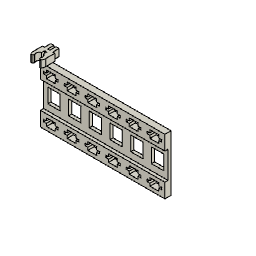
3mmビットホルダ v2 (Autodesk Fusion 360 design; units mm, degrees)
Autodesk Fusion 360 part; units mm, degrees
sketch "スケッチ1" plane through (0, 0, 0) normal (0, 0, 1) x (1, 0, 0)
  line L0 (-0.5, 1.519868) -> (-0.5, 3.5)
  line L1 (0.5, 3.5) -> (0.5, 1.519868)
  line L2 (-3, 0) -> (-3, 3.487815)
  line L3 (-1.811769, 6.5) -> (1.811769, 6.5)
  line L4 (3, 3.487815) -> (3, 0)
  line L5 (-0.5, 3.5) -> (0.5, 3.5)
  line L6 (1.02846, -1.225671) -> (1.928363, -2.298133)
  line L7 (0, 0) -> (3.962322, 0) construction
  line L8 (0, 0) -> (0, 0.7)
  line L9 (-1.02846, -1.225671) -> (-1.928363, -2.298133)
  arc A0 (-0.5, 1.519868) -> (-1.02846, -1.225671) centre (0, 0) ccw
  arc A1 (1.02846, -1.225671) -> (0.5, 1.519868) centre (0, 0) ccw
  arc A2 (-3, 0) -> (-1.928363, -2.298133) centre (0, 0) ccw
  arc A3 (1.928363, -2.298133) -> (3, 0) centre (0, 0) ccw
  line L10 (-1.811769, 3.487815) -> (-1.811769, 6.5)
  line L11 (1.811769, 3.487815) -> (1.811769, 6.5)
  line L12 (1.811769, 3.487815) -> (3, 3.487815)
  line L13 (-3, 3.487815) -> (-1.811769, 3.487815)
  line L14 (-0.5, 3.487815) -> (0.5, 3.487815)
  dimension "d1" = 3.2
  dimension "d4" = 6
  dimension "d6" = 50
  constraint coincident L7.start L8.start
  constraint concentric A0 A2
  constraint tangent L2 A2
  constraint perpendicular L2 L3
  constraint tangent L4 A2
  constraint perpendicular L3 L4
  constraint perpendicular L1 L5
  constraint horizontal L7
  constraint perpendicular L7 L8
  constraint concentric A0 A1
  constraint concentric A2 A3
  constraint perpendicular L4 L13
  constraint perpendicular L3 L10
  constraint collinear L12 L13
  constraint collinear L13 L14
  measures "d1" diameter of A0
  measures "d4" diameter of A2
  measures "d6" angle of L6 L7
extrude "押し出し1" add sketch "スケッチ1" along normal blind 3 contours L0 L1 L2 L3 L4 L5 L6 L9 A0 A1 A2 A3 L10 L11 L12 L13 picked at (0.166667, 5.5) makes body 1
sketch "スケッチ2" plane through (0, 6.5, 0) normal (0, 1, 0) x (-1, 0, 0)
  line L0 (-1.811769, 0) -> (1.811769, 0)
  line L1 (1.811769, 0) -> (1.811769, 3)
  line L2 (1.811769, 3) -> (-1.811769, 3)
  line L3 (-1.811769, 3) -> (-1.811769, 0)
  line L4 (-5, -2.005016) -> (5, -2.005016)
  line L5 (5, -2.005016) -> (5, 5)
  line L6 (5, 5) -> (-5, 5)
  line L7 (-5, 5) -> (-5, -2.005016)
  constraint horizontal L4
  constraint vertical L5
  constraint horizontal L6
  constraint vertical L7
extrude "押し出し2" add sketch "スケッチ2" against normal blind 3 separate body contours L4 L5 L6 L7 picked at (-3.937256, 0.998328) makes body 2
copy_body "ボディのコピーと貼り付け1" bodies 2 makes body 3
move_body "移動1" bodies 3 to x (1, 0, 0) y (0, 1, 0) z (0, 0, 1) at (0, 0, -30)
delete_body "RemoveBody1" bodies 3
move_face "面を移動1" by (0, 0, 0.3) 1 faces at (0.603923, 4.5, 3) on bodies 2
move_face "面を移動2" by (0.3, 0, 0) 1 faces at (1.811769, 5.5, 2.2) on bodies 2
move_face "面を移動3" by (-0.3, 0, 0) 1 faces at (-1.811769, 5.5, 1.1) on bodies 2
move_face "面を移動4" by (0, 0, -0.3) 1 faces at (0.703923, 5.5, 0) on bodies 2
sketch "スケッチ3" plane through (0, 6.5, 0) normal (0, 1, 0) x (-1, 0, 0)
  line L0 (-2.111769, -0.3) -> (-2.111769, 3.3)
  line L1 (-2.111769, 3.3) -> (2.111769, 3.3)
  line L2 (2.111769, 3.3) -> (2.111769, -0.3)
  line L3 (2.111769, -0.3) -> (-2.111769, -0.3)
  line L4 (-5, 5) -> (-5, -2.005016)
  line L5 (-5, -2.005016) -> (5, -2.005016)
  line L6 (5, -2.005016) -> (5, 5)
  line L7 (5, 5) -> (-5, 5)
  line L8 (3.5, 1) -> (-3.5, 1)
  line L9 (-3.5, 1) -> (-3.5, 2)
  line L10 (-3.5, 2) -> (3.5, 2)
  line L11 (3.5, 2) -> (3.5, 1)
  line L12 (3.5, 1) -> (-3.5, 2) construction
  line L13 (-3.5, 1) -> (3.5, 2) construction
  point P0 (0, 1.5)
  dimension "d11" = 7
  dimension "d12" = 1
  constraint horizontal L8
  constraint perpendicular L8 L9
  constraint parallel L8 L10
  constraint parallel L9 L11
  constraint coincident L12 P0
  constraint coincident L13 P0
  measures "d11" distance of L9.end L10.end
  measures "d12" distance of L8.end L9.end
extrude "押し出し3" cut sketch "スケッチ3" against normal blind 3.7 contours L0 L8 L9 L10 | L2 L8 L10 L11 picked at (-2.574513, 1.333333) picked at (2.574513, 1.666667) bodies 2
copy_body "ボディのコピーと貼り付け2" bodies 2 makes body 4
move_body "移動2" bodies 4 to x (1, 0, 0) y (0, 1, 0) z (0, 0, 1) at (0, 0, -30)
sketch "スケッチ4" plane through (0, 0, -2.005016) normal (0, 0, -1) x (1, 0, 0)
  line L0 (-5, -6.5) -> (5, -6.5)
  line L1 (5, -6.5) -> (5, -3.5)
  line L2 (5, -3.5) -> (-5, -3.5)
  line L3 (-5, -3.5) -> (-5, -6.5)
  line L4 (-5, -5) -> (5, -5)
  constraint midpoint L3 L4.start
  constraint midpoint L1 L4.end
extrude "押し出し4" add sketch "スケッチ4" along normal blind 23 contours L0 L1 L3 L4 picked at (-1.666667, -5.5) bodies 4 2
sketch "スケッチ5" plane through (0, 5, 0) normal (0, -1, 0) x (1, 0, 0)
  line L0 (-5, -25) -> (5, -25)
  line L1 (5, -25) -> (5, -2.005016)
  line L2 (5, -2.005016) -> (-5, -2.005016)
  line L3 (-5, -2.005016) -> (-5, -25)
  line L4 (2, -22) -> (-1.910963, -22)
  line L5 (-1.910963, -22) -> (-1.910963, -5.005015)
  line L6 (-1.910963, -5.005015) -> (2, -5.005015)
  line L7 (2, -5.005015) -> (2, -22)
  line L8 (2, -22) -> (-1.910963, -5.005015) construction
  line L9 (-1.910963, -22) -> (2, -5.005015) construction
  point P0 (0.044518, -13.502508)
  constraint horizontal L4
  constraint perpendicular L4 L5
  constraint parallel L4 L6
  constraint parallel L5 L7
extrude "押し出し5" cut sketch "スケッチ5" against normal blind 6 contours L4 L5 L6 L7 picked at (0.696346, -16.335005) bodies 4
move_face "面を移動5" by (0, 2, 0) 3 faces at (0.603923, 6.5, 2) (2.207846, 3.487815, 1) (-2.603923, 3.487815, 1) on bodies 1
move_body "移動3" bodies 1 to x (1, 0, 0) y (0, 1, 0) z (0, 0, 1) at (0, -2, 0)
move_face "面を移動6" by (1, 0, 0) 1 faces at (5, 5, -29.67001) on bodies 4
move_face "面を移動7" by (-1, 0, 0) 1 faces at (-5, 5, -29.67001) on bodies 4
move_face "面を移動8" by (-1, 0, 0) 1 faces at (-1.910963, 5.5, -16.335005) on bodies 4
move_face "面を移動9" by (1, 0, 0) 1 faces at (2, 6, -10.67001) on bodies 4
pattern_linear "R パターン1" count 1 spacing 0 along (0, 0, -1) count 6 spacing 12 along (1, 0, 0) of bodies 4 makes body 5 at (12.733602, 6.5, -3.436677) makes body 6 at (24.733602, 6.5, -3.436677) makes body 7 at (36.733602, 6.5, -3.436677) makes body 8 at (48.733602, 6.5, -3.436677) makes body 9 at (60.733602, 6.5, -3.436677)
combine "結合1" operation add target body 4 tool bodies 5 6 7 8 9
copy_body "ボディのコピーと貼り付け3" bodies 4 makes body 10
move_body "移動4" bodies 10 to x (1, 0, 0) y (0, 1, 0) z (0, 0, 1) at (75, 0, 0)
ref_plane "作業平面1" through (81.089037, 5.75, -13.502508) normal (1, 0, 0) x (0, 0, -1)
split "分割1" by plane through (81.089037, 5.75, -13.502508) normal (1, 0, 0) bodies 10 makes body 11 at (92.029679, 6.5, -10.67001)
sketch "スケッチ6" plane through (0, 0, 3) normal (0, 0, 1) x (-1, 0, 0)
  arc A0 (3, 2) -> (1.928363, 4.298133) centre (0, 2) ccw
  line L0 (1.928363, 4.298133) -> (1.02846, 3.225671)
  arc A1 (0.5, 0.480132) -> (1.02846, 3.225671) centre (0, 2) ccw
  line L1 (0.5, 0.480132) -> (0.5, -1.5)
  line L2 (0.5, -1.5) -> (-0.5, -1.5)
  line L3 (-0.5, -1.5) -> (-0.5, 0.480132)
  arc A2 (-1.02846, 3.225671) -> (-0.5, 0.480132) centre (0, 2) ccw
  line L4 (-1.02846, 3.225671) -> (-1.928363, 4.298133)
  arc A3 (-1.928363, 4.298133) -> (-3, 2) centre (0, 2) ccw
  line L5 (-3, 2) -> (-3, -3.487815)
  line L6 (-3, -3.487815) -> (-1.811769, -3.487815)
  line L7 (-1.811769, -3.487815) -> (-1.811769, -6.5)
  line L8 (-1.811769, -6.5) -> (1.811769, -6.5)
  line L9 (1.811769, -6.5) -> (1.811769, -3.487815)
  line L10 (1.811769, -3.487815) -> (3, -3.487815)
  line L11 (3, -3.487815) -> (3, 2)
  line L12 (-0.5, -3.5) -> (0.5, -3.5)
  line L13 (0.5, -3.5) -> (0.5, -9.5)
  line L14 (0.5, -9.5) -> (-0.5, -9.5)
  line L15 (-0.5, -9.5) -> (-0.5, -3.5)
  line L16 (-0.5, -3.5) -> (0.5, -9.5) construction
  line L17 (0.5, -3.5) -> (-0.5, -9.5) construction
  point P0 (0, -6.5)
  constraint horizontal L12
  constraint perpendicular L12 L13
  constraint parallel L12 L14
  constraint parallel L13 L15
  constraint coincident L16 P0
  constraint coincident L17 P0
  constraint midpoint L8 P0
extrude "押し出し6" cut sketch "スケッチ6" against normal blind 6 contours L8 L12 L13 L15 picked at (-0.166667, -4.5) bodies 1
move_body "移動5" bodies 10 to x (1, 0, 0) y (0, 1, 0) z (0, 0, 1) at (-75, 0, 0)
move_face "面を移動10" by (1, 0, 0) 1 faces at (-6, 5, -29.67001) on bodies 10
move_face "面を移動11" by (-1, 0, 0) 1 faces at (6.089037, 5, -29.67001) on bodies 10
copy_body "ボディのコピーと貼り付け4" bodies 10 makes body 12
pattern_linear "R パターン2" count 6 spacing 10 along (1, 0, 0) of bodies 12 makes body 13 at (10.733602, 6.5, -3.436677) makes body 14 at (20.733602, 6.5, -3.436677) makes body 15 at (30.733602, 6.5, -3.436677) makes body 16 at (40.733602, 6.5, -3.436677) makes body 17 at (50.733602, 6.5, -3.436677)
combine "結合2" operation add target body 17 tool bodies 16 15 14 12 13
move_face "面を移動12" by (0.229813, 0.192836, 0) 1 faces at (1.328428, -3.583159, 1) on bodies 1
move_face "面を移動13" by (-0.229813, 0.192836, 0) 1 faces at (-1.328428, -3.583159, 1) on bodies 1
move_face "面を移動14" by (-0.3, 0, 0) 1 faces at (-1.811769, 4.491877, 1) on bodies 1
move_face "面を移動15" by (0.3, 0, 0) 1 faces at (1.811769, 4.491877, 1) on bodies 1
move_face "面を移動16" by (0, 0, 0.4) 1 faces at (-2.422319, 0.154988, 3) on bodies 1
chamfer "面取り1" distance 0.2 angle 45 2 edges at (1.240033, -3.011097, 1.7) (-1.240033, -3.011097, 1.7) on bodies 1
chamfer "面取り2" distance 0.5 angle 45 2 edges at (2.14851, -4.093778, 1.7) (-2.14851, -4.093778, 1.7) on bodies 1
move_face "面を移動17" by (-0.1, 0, 0) 1 faces at (2.111769, 4.491877, 1.133333) on bodies 1
move_face "面を移動18" by (0.1, 0, 0) 1 faces at (-2.111769, 4.491877, 1.133333) on bodies 1
ref_plane "作業平面2" through (25.044518, 5, -13) normal (0, 0, 1) x (-1, 0, 0)
split "分割2" by plane through (25.044518, 5, -13) normal (0, 0, 1) bodies 17 makes body 18 at (0.733602, 6.5, -3.436677)
move_body "移動6" bodies 18 to x (1, 0, 0) y (0, 1, 0) z (0, 0, 1) at (0, 0, -10)
combine "結合3" operation add target body 17 tool bodies 18
delete_body "RemoveBody2" bodies 11
delete_body "RemoveBody3" bodies 4
delete_body "RemoveBody4" bodies 10
move_face "面を移動19" by (0, -1, 0) 5 faces at (1.003923, 6.5, 1.133333) (-1.507846, 6.5, 1.133333) (-0.166667, 3.5, 1.133333) (2.34118, 3.487815, 1.133333) (-2.67059, 3.487815, 1.133333) on bodies 1
move_face "面を移動20" by (0, -0.5, 0) 1 faces at (-0.166667, 1.5, 1.133333) on bodies 1
named bodies: "クリップ", "Umderx6_", "Umder", "Umder x1_", "Umderx5_", "Umder x1_ (1)", "Umder x1_ (1) (1)", "Umder x1_ (1) (2)", "Umder x1_ (1) (3)", "Umder x1_ (1) (4)", "Umder x6", "Umder x6_ b (1)"
